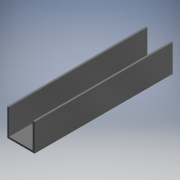
# Autodesk Inventor part: Claw holding bars
Saved by Autodesk Inventor 2019 (Build 230136000, 136)
## iProperties
Part Number: Claw holding bars
Material: Generic
Document SubType Name: Modeling
Designer: Delta
Appearance: Default
Author: Delta
Autodesk Inventor part; units mm, degrees
ref_plane "YZ Plane" through (0, 0, 0) normal (1, 0, 0) x (0, 1, 0)
ref_plane "XZ Plane" through (0, 0, 0) normal (0, 1, 0) x (-1, 0, 0)
ref_plane "XY Plane" through (0, 0, 0) normal (0, 0, 1) x (1, 0, 0)
sketch "Sketch1" plane through (0, 0, 0) normal (0, 0, 1) x (1, 0, 0)
  line L0 (0, 0) -> (31.75, 0)
  line L1 (31.75, 0) -> (31.75, 31.75)
  line L2 (31.75, 31.75) -> (0, 31.75)
  line L3 (0, 31.75) -> (0, 0)
  dimension "d0" = 31.75
  dimension "d1" = 31.75
  constraints: 8 end point, 2 parallel, 1 horizontal, 1 perpendicular
  measures "d0" distance of L2.end L1.end
  measures "d1" distance between parallel lines of L0 L2
extrude "Extrusion1" add sketch "Sketch1" along normal blind 160.3375
sketch "Sketch2" plane through (0, 0, 160.3375) normal (0, 0, 1) x (1, 0, 0)
  circle A0 centre (15.875, 15.875) radius 2.54
  line L0 (31.75, 31.75) -> (0, 31.75) projected
  line L1 (0, 0) -> (31.75, 0) projected
  line L2 (0, 31.75) -> (0, 0) projected
  dimension "d4" = 5.08
  dimension "d5" = 31.75
  dimension "d6" = 15.875
  dimension "d7" = 15.875
  constraints: 1 centre point
  measures "d4" diameter of A0
  measures "d5" distance between parallel lines of L0 L1
  measures "d6" distance from line of L2 A0.centre
  measures "d7" distance from line of L0 A0.centre
extrude "Extrusion2" cut sketch "Sketch2" against normal through all
sketch "Sketch3" plane through (0, 31.75, 0) normal (0, 1, 0) x (1, 0, 0)
  line L0 (31.75, 0) -> (0, 0) projected
  line L1 (0, 0) -> (0, -160.3375) projected
  line L2 (31.75, 0) -> (31.75, -160.3375) projected
  line L3 (31.75, -160.3375) -> (0, -160.3375) projected
  line L4 (2.032, 0) -> (29.718, 0)
  line L5 (29.718, 0) -> (29.718, -160.3375)
  line L6 (29.718, -160.3375) -> (2.032, -160.3375)
  line L7 (2.032, -160.3375) -> (2.032, 0)
  dimension "d10" = 0
  dimension "d11" = 2.032
  dimension "d12" = 2.032
  dimension "d13" = 0
  constraints: 8 end point, 2 parallel, 1 horizontal, 1 perpendicular
  measures "d10" distance from line of L0 L4.start
  measures "d11" distance from line of L1 L4.start
  measures "d12" distance from line of L2 L5.end
  measures "d13" distance from line of L3 L5.end
extrude "Extrusion3" cut sketch "Sketch3" against normal blind 29.718 contours L5 L3 L7 L0
equation "\"d1\" = d0"
equation "\"d6\" = 0.5 * d5"
equation "\"d7\" = d6"
equation "\"d12\" = d11"
body "Solid1"
